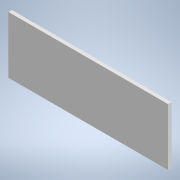
# Autodesk Inventor part: achterruit
Saved by Autodesk Inventor 2022 (Build 260153000, 153)
## iProperties
Created: 2021-12-16
Part Number: achterruit
Material: Generic
Document SubType Name: Modeling
Designer: keemi
Density: 1 g/cm^3
Appearance: Default
Author: keemi
Autodesk Inventor part; units mm, degrees
ref_plane "YZ Plane" through (0, 0, 0) normal (1, 0, 0) x (0, 1, 0)
ref_plane "XZ Plane" through (0, 0, 0) normal (0, 1, 0) x (-1, 0, 0)
ref_plane "XY Plane" through (0, 0, 0) normal (0, 0, 1) x (1, 0, 0)
sketch "Sketch1" plane through (0, 0, 0) normal (0, 0, 1) x (1, 0, 0)
  line L0 (0, 0) -> (-140, 0)
  line L1 (-140, 0) -> (-140, 40)
  line L2 (-140, 40) -> (0, 40)
  line L3 (0, 40) -> (0, 0)
  line L4 (-140, 0) -> (0, 0)
  line L5 (0, 0) -> (0, -10)
  line L6 (0, -10) -> (-140, -10)
  line L7 (-140, -10) -> (-140, 0)
  dimension "d0" = 140
  dimension "d1" = 40
  dimension "d2" = 10
  constraints: 16 end point, 4 parallel, 2 horizontal, 2 perpendicular
  measures "d0" distance of L1.end L2.end
  measures "d1" distance of L0.end L1.end
  measures "d2" distance of L4.end L5.end
extrude "Extrusion1" add sketch "Sketch1" against normal blind 3
body "Solid1"
